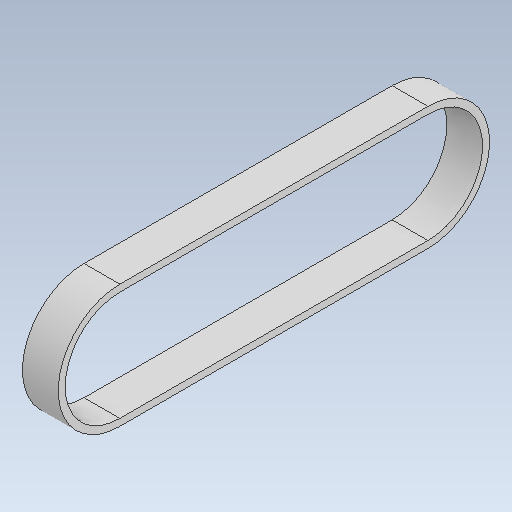
# Autodesk Inventor part: 49T belt from gobuilda
Saved by Autodesk Inventor 2020.2 (Build 242310000, 310)
## iProperties
Created: 2020-03-01
Part Number: 49T belt from gobuilda
Material: Generic
Document SubType Name: Modeling
Designer: deli
Density: 1 g/cm^3
Appearance: Default
Author: deli
Autodesk Inventor part; units mm, degrees
ref_plane "YZ Plane" through (0, 0, 0) normal (1, 0, 0) x (0, 1, 0)
ref_plane "XZ Plane" through (0, 0, 0) normal (0, 1, 0) x (-1, 0, 0)
ref_plane "XY Plane" through (0, 0, 0) normal (0, 0, 1) x (1, 0, 0)
sketch "Sketch1" plane through (0, 0, 0) normal (1, 0, 0) x (0, 1, 0)
  arc A0 (7.1618, 41.4339) -> (-20.3375, 41.4339) centre (-6.5878, 41.4339) ccw
  arc A1 (-20.3375, -36.0661) -> (7.1618, -36.0661) centre (-6.5878, -36.0661) ccw
  line L0 (7.1618, 41.4339) -> (7.1618, -36.0661)
  line L1 (-20.3375, -36.0661) -> (-20.3375, 41.4339)
  line L2 (8.9018, -36.0661) -> (8.9018, 41.4339)
  arc A2 (8.9018, 41.4339) -> (-22.0775, 41.4339) centre (-6.5878, 41.4339) ccw
  line L3 (-22.0775, 41.4339) -> (-22.0775, -36.0661)
  arc A3 (-22.0775, -36.0661) -> (8.9018, -36.0661) centre (-6.5878, -36.0661) ccw
  point P0 (0, 0)
  dimension "d0" = 27.4993
  dimension "d1" = 27.4993
  dimension "d2" = 77.5
  dimension "d3" = 0
  dimension "d4" = 1.74
  constraints: 8 end point, 8 point on circle, 4 centre point, 1 tangent, 1 vertical, 3 other
  measures "d0" diameter of A0
  measures "d1" diameter of A1
  measures "d2" distance of A1.centre A0.centre
  measures "d3" horizontal distance of A1.centre A0.centre
  measures "d4" distance between parallel lines of L0 L2
extrude "Extrusion1" add sketch "Sketch1" along normal blind 9
equation "\"d1\" = d0"
body "Solid1"
